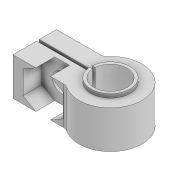
# Autodesk Inventor part: Clamping Collar 1_4
Saved by Autodesk Inventor 2020 (Build 240168000, 168)
## iProperties
Created: 2019-11-09
Part Number: Clamping Collar 1_4
Material: Generic
Document SubType Name: Modeling
Designer: ball
Density: 1 g/cm^3
Appearance: Default
Author: ball
Autodesk Inventor part; units mm, degrees
ref_plane "YZ Plane" through (0, 0, 0) normal (1, 0, 0) x (0, 1, 0)
ref_plane "XZ Plane" through (0, 0, 0) normal (0, 1, 0) x (-1, 0, 0)
ref_plane "XY Plane" through (0, 0, 0) normal (0, 0, 1) x (1, 0, 0)
sketch "Sketch1" plane through (0, 0, 0) normal (0, 1, 0) x (-1, 0, 0)
  arc A0 (3.8932, 5.0165) -> (5.127, -3.7465) centre (0, 0) ccw
  arc A1 (3.3559, 0.254) -> (3.3559, -0.254) centre (0, 0) ccw
  line L0 (14.605, -0.254) -> (14.605, -3.7465)
  line L1 (14.605, -3.7465) -> (5.127, -3.7465)
  line L2 (14.605, 0.254) -> (14.605, 5.0165)
  line L3 (14.605, 5.0165) -> (3.8932, 5.0165)
  line L4 (3.3559, -0.254) -> (14.605, -0.254)
  line L5 (3.3559, 0.254) -> (14.605, 0.254)
  dimension "d0" = 12.7
  dimension "d1" = 6.731
  dimension "d8" = 0.254
  dimension "d9" = 0.254
  dimension "d10" = 4.7625
  dimension "d11" = 3.4925
  dimension "d25" = 14.605
  dimension "d26" = 14.605
  constraints: 12 end point, 4 point on circle, 2 centre point, 2 coincident
  measures "d0" diameter of A0
  measures "d1" diameter of A1
  measures "d8" distance from line of L5 point (0, 0)
  measures "d9" distance from line of L4 point (0, 0)
  measures "d10" distance between parallel lines of L3 L5
  measures "d11" distance between parallel lines of L1 L4
  measures "d25" distance from line of L2 point (0, 0)
  measures "d26" distance from line of L0 point (0, 0)
extrude "PartThickness" add sketch "Sketch1" along normal blind 7.62
sketch "Sketch2" plane through (0, 7.62, 0) normal (0, 1, 0) x (1, 0, 0)
  arc A0 (-3.9288, -0.254) -> (-3.9288, 0.254) centre (0, 0) ccw
  arc A1 (-3.3559, -0.254) -> (-3.3559, 0.254) centre (0, 0) ccw
  line L0 (-3.3559, -0.254) -> (-14.605, -0.254) projected
  line L1 (-3.9288, -0.254) -> (-3.3559, -0.254)
  line L2 (-14.605, 0.254) -> (-3.3559, 0.254) projected
  arc A2 (-3.3559, -0.254) -> (-3.3559, 0.254) centre (0, 0) ccw projected
  line L3 (-14.605, 0.254) -> (-3.3559, 0.254) projected
  line L4 (-3.9288, 0.254) -> (-3.3559, 0.254)
  dimension "d14" = 7.874
  constraints: 4 end point, 4 point on circle, 3 point on line, 2 centre point, 2 coincident, 2 collinear
  measures "d14" diameter of A0
extrude "RaceStandoff" add sketch "Sketch2" along normal blind 0.762
sketch "Sketch3" plane through (-14.605, 0, 5.0165) normal (0, 0, 1) x (1, 0, 0)
  line L0 (0, 0) -> (0, 7.62) construction
  line L1 (0, 3.81) -> (11.9818, 3.81) construction
  line L2 (10.7118, 0) -> (10.7118, 7.62) construction
  circle A0 centre (6.0509, 3.81) radius 4.6609 construction
  line L3 (6.0509, -0.8509) -> (2.0144, 1.4796)
  line L4 (2.0144, 1.4796) -> (2.0144, 6.1404)
  line L5 (2.0144, 6.1404) -> (6.0509, 8.4709)
  line L6 (6.0509, 8.4709) -> (10.0873, 6.1405)
  line L7 (10.0873, 6.1405) -> (10.0873, 1.4796)
  line L8 (10.0873, 1.4796) -> (6.0509, -0.8509)
  point P0 (14.605, 0)
  dimension "d18" = 9.3218
  dimension "d19" = 4.6609
  constraints: 14 end point, 2 coincident, 1 midpoint, 1 point on line, 1 vertical alignment, 16 other
  measures "d19" distance from line of L2 point (6.051, 3.81)
extrude "NutWell" cut sketch "Sketch3" against normal blind 3.81
sketch "Sketch4" plane through (-14.605, 0, 1.2065) normal (0, 0, 1) x (1, 0, 0)
  line L0 (10.7118, 0) -> (10.7118, 7.62) construction
  line L1 (10.6762, 7.62) -> (0, 7.62) construction
  circle A0 centre (6.0509, 3.81) radius 1.9304
  line L2 (2.0144, 6.1404) -> (4.5771, 7.62) construction
  line L3 (10.0873, 6.1405) -> (10.0873, 1.4796) construction
  line L4 (2.0144, 6.1404) -> (10.0873, 1.4796) construction
  line L5 (10.0873, 1.4796) -> (10.0873, 6.1404) construction
  line L6 (4.5771, 0) -> (2.0144, 1.4796) construction
  line L7 (10.0873, 6.1404) -> (2.0144, 1.4796) construction
  point P0 (14.605, 0)
  point P1 (11.9818, 3.81)
  point P2 (12.5191, 7.62)
  dimension "d22" = 3.8608
  constraints: 6 end point, 1 centre point, 1 coincident, 1 midpoint, 1 other
  measures "d22" diameter of A0
extrude "ScrewHole" cut sketch "Sketch4" against normal through all
fillet "Fillet1" radius 1.27 1 edges at (-5.127, 3.81, -3.7465)
fillet "Fillet2" radius 1.778 1 edges at (-3.8932, 3.81, 5.0165)
body "Solid1"
